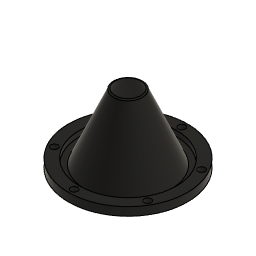
筒固定具 (Autodesk Fusion 360 design; units mm, degrees)
Autodesk Fusion 360 part; units mm, degrees
note: some values were not read from the file. Set by a fixed rule: which sketch regions a step uses.
sketch "スケッチ1" plane through (0, 0, 0) normal (0, 0, 1) x (1, 0, 0)
  circle A0 centre (0, 0) radius 17.5
  circle A1 centre (0, 0) radius 23.5
  line L0 (0, 0) -> (0, 23.5)
  circle A2 centre (0, 20.5) radius 1.5
  circle A3 centre (-17.7535, 10.25) radius 1.5
  circle A4 centre (-17.7535, -10.25) radius 1.5
  circle A5 centre (0, -20.5) radius 1.5
  circle A6 centre (17.7535, -10.25) radius 1.5
  circle A7 centre (17.7535, 10.25) radius 1.5
  dimension "d1" = 35
  dimension "d2" = 47
  dimension "d4" = 360
  constraint coincident A0.centre A1.centre
  constraint coincident A1 L0.end
  constraint vertical L0
  constraint coincident L0 A2.centre
  measures "d1" diameter of A0
  measures "d2" diameter of A1
extrude "押し出し1" add sketch "スケッチ1" along normal blind 3
sketch "スケッチ2" plane through (0, 0, 3) normal (0, 0, 1) x (-1, 0, 0)
  circle A0 centre (0, 0) radius 17.5
  circle A1 centre (17.7535, -10.25) radius 1.5
  circle A2 centre (0, -20.5) radius 1.5
  circle A3 centre (17.7535, 10.25) radius 1.5
  circle A4 centre (0, 20.5) radius 1.5
  circle A5 centre (-17.7535, 10.25) radius 1.5
  circle A6 centre (-17.7535, -10.25) radius 1.5
  circle A7 centre (0, 0) radius 23.5
extrude "押し出し2" add sketch "スケッチ2" against normal blind 3 contours A1 | A2 | A3 | A4 | A5 | A6
sketch "スケッチ3" plane through (0, 0, 3) normal (0, 0, 1) x (-1, 0, 0)
  circle A0 centre (0, 0) radius 17.5
  circle A1 centre (0, 0) radius 23.5
  circle A2 centre (0, 0) radius 21.5
  dimension "d9" = 43
  constraint concentric A0 A2
  measures "d9" diameter of A2
extrude "押し出し3" cut sketch "スケッチ3" against normal blind 19 contours A1
sketch "スケッチ4" plane through (0, 0, 3) normal (0, 0, 1) x (-1, 0, 0)
  circle A0 centre (0, 0) radius 21.5
  circle A1 centre (0, 0) radius 17.5
  line L0 (0, 22) -> (0, 17)
  line L1 (0, 17.5) -> (0, 21.5)
  circle A2 centre (0, 19.5) radius 1.25
  circle A3 centre (-16.8875, 9.75) radius 1.25
  circle A4 centre (-16.8875, -9.75) radius 1.25
  circle A5 centre (0, -19.5) radius 1.25
  circle A6 centre (16.8875, -9.75) radius 1.25
  circle A7 centre (16.8875, 9.75) radius 1.25
  dimension "d12" = 2.5
  dimension "d14" = 360
  constraint vertical L0
  constraint coincident L0 L1.start
  constraint coincident A1 L1.start
  constraint coincident L0 L1.end
  constraint coincident A0 L1.end
  constraint midpoint L1 A2.centre
  measures "d12" diameter of A2
extrude "押し出し4" cut sketch "スケッチ4" against normal blind 10 contours L0 L1 A2 | L0 L1 A2 | A3 | A4 | A5 | A6 | A7
sketch "スケッチ5" plane through (0, 0, 0) normal (0, 0, 1) x (1, 0, 0)
  circle A0 centre (0, 0) radius 17.5
  circle A1 centre (0, 0) radius 15.5
  dimension "d17" = 31
  constraint coincident A0.centre A1.centre
  measures "d17" diameter of A1
extrude "押し出し5" add sketch "スケッチ5" along normal blind 1
sketch "スケッチ6" plane through (0, 0, 0) normal (0, 1, 0) x (1, 0, 0)
  line L0 (-15.5, -3.5) -> (-15.5, 1.5)
  line L1 (-15.5, 0) -> (-15.5, -1)
  line L2 (-15.5, -1) -> (-15.5, -25.9)
  line L3 (0, -25.9) -> (4.631, -25.9)
  line L4 (0, -25.9) -> (-4.631, -25.9)
  line L5 (-15.5, -1) -> (-4.631, -25.9)
  line L6 (-15.5, 0) -> (-4.631, -24.9)
  line L7 (-4.631, -24.9) -> (-4.631, -25.9)
  dimension "d20" = 24.9
  dimension "d21" = 4.631
  dimension "d22" = 4.631
  constraint vertical L0
  constraint coincident L0 L1.start
  constraint midpoint L0 L1.end
  constraint parallel L0 L2
  constraint perpendicular L2 L3
  constraint parallel L3 L4
  constraint parallel L5 L6
  constraint perpendicular L4 L7
  measures "d20" distance of L1.end L2.end
  measures "d21" distance of L3.start L3.end
  measures "d22" distance of L3.start L4.end
revolve "回転1" add sketch "スケッチ6" angle 360 about axis through (0, 0, 1.75) along (0, 0, 1)
fillet "フィレット1" radius 0.5 1 edges at (-4.3176, 1.6746, 25.9)
fillet "フィレット2" radius 1 1 edges at (-14.4511, 5.605, 0)
